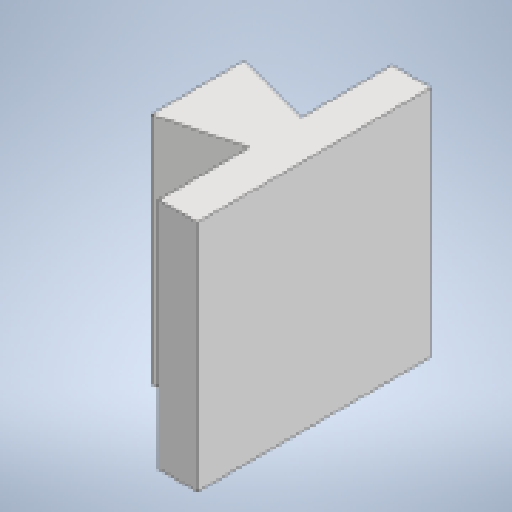
# Autodesk Inventor part: Laser_Mount
Saved by Autodesk Inventor 2023 (Build 270158000, 158)
## iProperties
Created: 2024-01-06
Part Number: Laser_Mount
Material: Generic
Document SubType Name: Modeling
Designer: a laptop
Density: 1 g/cm^3
Appearance: Default
Author: a laptop
Autodesk Inventor part; units mm, degrees
ref_plane "YZ Plane" through (0, 0, 0) normal (1, 0, 0) x (0, 1, 0)
ref_plane "XZ Plane" through (0, 0, 0) normal (0, 1, 0) x (-1, 0, 0)
ref_plane "XY Plane" through (0, 0, 0) normal (0, 0, 1) x (1, 0, 0)
sketch "Sketch1" plane through (0, 0, 0) normal (0, 1, 0) x (-1, 0, 0)
  line L0 (0, 0) -> (5, 0)
  line L1 (5, 0) -> (5, -11.6795)
  line L2 (5, -11.6795) -> (15, -9)
  line L3 (15, -9) -> (15, -21)
  line L4 (15, -21) -> (5, -18.3205)
  line L5 (5, -18.3205) -> (5, -30)
  line L6 (5, -30) -> (0, -30)
  line L7 (0, -30) -> (0, 0)
  dimension "d0" = 30
  dimension "d1" = 12
  dimension "d2" = 30
  dimension "d3" = 10
  dimension "d4" = 5
  constraints: 16 end point, 3 perpendicular, 2 equal length, 2 point on line, 1 horizontal, 1 parallel
  measures "d0" angle of L4 L2
  measures "d1" distance of L2.end L3.end
  measures "d2" distance of L6.end L0.start
  measures "d3" distance from line of L4.end L3
  measures "d4" distance of L5.end L6.end
extrude "Extrusion1" add sketch "Sketch1" along normal blind 30
body "Solid1"
